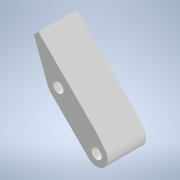
# Autodesk Inventor part: laser_krepl_right
Saved by Autodesk Inventor 2022 (Build 260153000, 153)
## iProperties
Created: 2023-01-26
Part Number: laser_krepl_right
Material: Типовые
Document SubType Name: Modeling
Designer: akapu
Density: 1 g/cm^3
Appearance: По умолчанию
Author: akapu
Autodesk Inventor part; units mm, degrees
ref_plane "YZ Plane" through (0, 0, 0) normal (1, 0, 0) x (0, 1, 0)
ref_plane "XZ Plane" through (0, 0, 0) normal (0, 1, 0) x (-1, 0, 0)
ref_plane "XY Plane" through (0, 0, 0) normal (0, 0, 1) x (1, 0, 0)
sketch "Эскиз1" plane through (0, 0, 0) normal (0, 0, 1) x (1, 0, 0)
  line L0 (-5, -1.0438) -> (49.0851, -1.0438) projected
  circle A0 centre (141.53, 31.3) radius 1.6
  circle A1 centre (141.53, 31.3) radius 12.8551
  line L1 (141.53, 31.3) -> (144.3584, 34.1284)
  line L2 (144.3584, 34.1284) -> (153.4483, 25.0385)
  line L3 (144.3584, 34.1284) -> (135.2685, 43.2183)
  line L4 (135.2685, 43.2183) -> (132.4401, 40.3899)
  line L5 (133.8543, 41.8041) -> (152.0341, 23.6243)
  line L6 (152.0341, 23.6243) -> (153.4483, 25.0385)
  circle A2 centre (141.53, 31.3) radius 3.5
  line L7 (133.8543, 41.8041) -> (138.2527, 30.0714)
  line L8 (141.53, 31.3) -> (150.6199, 22.2101)
  line L9 (150.6199, 22.2101) -> (153.4483, 19.3817)
  circle A3 centre (153.4483, 19.3817) radius 1.6
  circle A4 centre (153.4483, 19.3817) radius 3.5
  line L10 (139.0551, 28.8251) -> (150.9734, 16.9068)
  line L11 (153.4483, 25.0385) -> (156.198, 21.5472)
  ellipse E0 centre (50.75, 20.1064) end of major axis (50.75, -5.3184) minor radius 3 (49.0851, -1.0438) -> (50.4608, -5.2) ccw projected
  line L12 (-5, -9.3562) -> (-5, -1.0438) projected
  line L13 (49.0851, -9.3562) -> (-5, -9.3562) projected
  ellipse E1 centre (50.75, -30.5064) end of major axis (50.75, -5.0816) minor radius 3 (50.4608, -5.2) -> (49.0851, -9.3562) ccw projected
  line L14 (135.2688, -53.6185) -> (153.4482, -35.4383) projected
  line L15 (153.4482, -35.4383) -> (156.1979, -31.9467) projected
  arc A5 (156.1979, -31.9467) -> (150.9733, -27.3065) centre (153.4482, -29.7813) ccw projected
  line L16 (150.9733, -27.3065) -> (139.0551, -39.2252) projected
  arc A6 (139.0551, -39.2252) -> (138.2526, -40.4715) centre (141.5299, -41.7001) ccw projected
  line L17 (138.2526, -40.4715) -> (133.8546, -52.2043) projected
  line L18 (133.8546, -52.2043) -> (135.2688, -53.6185) projected
  circle A7 centre (153.4482, -29.7813) radius 1.6 projected
  circle A8 centre (141.5299, -41.7001) radius 1.6 projected
  arc A9 (133.5218, -22.9864) -> (138.03, -21.6481) centre (141.53, -41.7) ccw projected
  arc A10 (138.03, -25.2121) -> (137.4201, -25.3535) centre (141.5299, -41.7001) ccw projected
  line L19 (137.4201, -25.3535) -> (133.5218, -22.9864) projected
  line L20 (138.03, -21.6481) -> (138.03, -25.2121) projected
  point P0 (0, 0)
  point P1 (139.0604, -39.2199)
  point P2 (144.9752, 30.6832)
  point P3 (140.9132, 34.7452)
  point P4 (133.9107, 41.6537)
  point P5 (135.7198, 42.7671)
  dimension "d0" = 3.2
  dimension "d1" = 4
  dimension "d2" = 7
  dimension "d3" = 4
  dimension "d4" = 3.2
  dimension "d5" = 7
  constraints: 22 end point, 6 point on circle, 5 centre point, 4 coincident, 4 tangent, 3 perpendicular, 1 midpoint, 1 point on line, 2 other
  measures "d0" diameter of A0
  measures "d1" distance of L1.start L1.end
  measures "d2" diameter of A2
  measures "d3" distance of L8.end L9.end
  measures "d4" diameter of A3
  measures "d5" diameter of A4
extrude "Выдавливание1" add sketch "Эскиз1" against normal blind 12 contours A0 L1 L5 A2 L8 | A0 L8 A2 L5 L1 | L5 A2 L1 | L1 A2 L5 | L8 A1 L10 A2 | A2 L5 A1 L8 | A2 L5 A1 L3 L1 | L1 L2 A1 L5 A2 | A2 L7 A1 L5 | L9 A4 L10 A1 | A1 L5 L6 L11 A4 L9 | L5 L4 L3 A1 | A1 L7 L5 | A1 L2 L6 L5 | A4
chamfer "Фаска1" distance 1 angle 45 2 edges at (151.8483, 19.3817, -12) (139.93, 31.3, -12)
sketch "Эскиз2" plane through (153.4483, 25.0385, 0) normal (0.7071068, 0.7071068, 0) x (0, 0, -1)
  line L0 (0, 25.7101) -> (12, 25.7101) projected
  line L1 (6, 25.7101) -> (6, 21.4051)
  line L2 (6, 21.4051) -> (6, -7.5)
  line L3 (0, -7.5) -> (12, -7.5) projected
  line L4 (6, 21.4051) -> (6, 1.9051)
  circle A0 centre (6, 21.4051) radius 1.6
  circle A1 centre (6, 1.9051) radius 1.6
  point P0 (0, 90.7994)
  dimension "d11" = 4.305
  dimension "d12" = 19.5
  dimension "d13" = 3.2
  dimension "d14" = 3.2
  constraints: 6 end point, 2 centre point, 2 coincident, 2 midpoint, 1 point on line, 1 vertical
  measures "d11" distance of L1.start L1.end
  measures "d12" distance of L1.end L4.end
  measures "d13" diameter of A0
  measures "d14" diameter of A1
extrude "Выдавливание2" [suppressed]
chamfer "Фаска2" [suppressed]
sketch "Эскиз3" plane through (139.0551, 28.8251, -12) normal (-0.7071068, -0.7071068, 0) x (0, 0, 1)
  circle A0 centre (6, -10.9499) radius 1.6 projected
  line L0 (6, -10.9499) -> (8.7, -10.9499)
  line L1 (8.7, -12.5088) -> (6, -14.0676)
  line L2 (6, -14.0676) -> (3.3, -12.5088)
  line L3 (3.3, -12.5088) -> (3.3, -9.3911)
  line L4 (3.3, -9.3911) -> (6, -7.8323)
  line L5 (6, -7.8323) -> (8.7, -9.3911)
  line L6 (8.7, -9.3911) -> (8.7, -12.5088)
  point P0 (12, 77.9444)
  dimension "d20" = 2.7
  constraints: 14 end point, 1 coincident, 1 horizontal, 1 midpoint, 13 other
  measures "d20" distance of L0.start L0.end
extrude "Выдавливание3" cut sketch "Эскиз3" against normal blind 1.5
sketch "Эскиз4" plane through (139.0551, 28.8251, -12) normal (-0.7071068, -0.7071068, 0) x (0, 0, 1)
  circle A0 centre (6, 8.5501) radius 1.6 projected
  line L0 (6, 8.5501) -> (8.7, 8.5501)
  line L1 (12, -12.8551) -> (12, 12.2169) projected
  line L2 (8.7, 6.9912) -> (6, 5.4324)
  line L3 (6, 5.4324) -> (3.3, 6.9912)
  line L4 (3.3, 6.9912) -> (3.3, 10.1089)
  line L5 (3.3, 10.1089) -> (6, 11.6677)
  line L6 (6, 11.6677) -> (8.7, 10.1089)
  line L7 (8.7, 10.1089) -> (8.7, 6.9912)
  point P0 (12, 77.9444)
  point P1 (12, 12.8551)
  point P2 (6, 8.5501)
  dimension "d23" = 2.7
  constraints: 14 end point, 1 coincident, 1 midpoint, 1 perpendicular, 13 other
  measures "d23" distance of L0.start L0.end
extrude "Выдавливание4" cut sketch "Эскиз4" against normal blind 5
